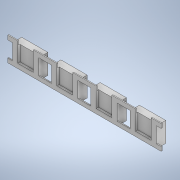
# Autodesk Inventor part: buttons
Saved by Autodesk Inventor 2020 (Build 240168000, 168)
## iProperties
Created: 2022-10-02
Part Number: buttons
Material: Типовые
Document SubType Name: Modeling
Designer: NoName
Density: 1 g/cm^3
Appearance: По умолчанию
Author: NoName
Autodesk Inventor part; units mm, degrees
ref_plane "YZ Plane" through (0, 0, 0) normal (1, 0, 0) x (0, 1, 0)
ref_plane "XZ Plane" through (0, 0, 0) normal (0, 1, 0) x (-1, 0, 0)
ref_plane "XY Plane" through (0, 0, 0) normal (0, 0, 1) x (1, 0, 0)
sketch "Эскиз1" plane through (0, 0, 0) normal (0, 0, 1) x (1, 0, 0)
  line L0 (0, 0) -> (5.7, 0)
  line L1 (5.7, 0) -> (5.7, 4.3)
  line L2 (5.7, 4.3) -> (0, 4.3)
  line L3 (0, 4.3) -> (0, 0)
  line L4 (8.5, 0) -> (14.2, 0)
  line L5 (14.2, 0) -> (14.2, 4.3)
  line L6 (14.2, 4.3) -> (8.5, 4.3)
  line L7 (8.5, 4.3) -> (8.5, 0)
  line L8 (17, 0) -> (22.7, 0)
  line L9 (22.7, 0) -> (22.7, 4.3)
  line L10 (22.7, 4.3) -> (17, 4.3)
  line L11 (17, 4.3) -> (17, 0)
  line L12 (25.5, 0) -> (31.2, 0)
  line L13 (31.2, 0) -> (31.2, 4.3)
  line L14 (31.2, 4.3) -> (25.5, 4.3)
  line L15 (25.5, 4.3) -> (25.5, 0)
  dimension "d0" = 4.3
  dimension "d1" = 5.7
  dimension "d4" = 8.5
  constraints: 32 end point, 2 horizontal, 2 parallel, 1 collinear, 1 perpendicular, 23 other
  measures "d0" distance between parallel lines of L0 L2
  measures "d1" distance between parallel lines of L1 L3
  measures "d4" distance of L0.start L4.start
extrude "Выдавливание1" add sketch "Эскиз1" along normal blind 2.4
sketch "Эскиз2" plane through (0, 0, 2.4) normal (0, 0, 1) x (1, 0, 0)
  line L0 (-1, 4.3) -> (32.2, 4.3)
  line L1 (32.2, 4.3) -> (32.2, 5.2)
  line L2 (32.2, 5.2) -> (-1, 5.2)
  line L3 (-1, 5.2) -> (-1, 4.3)
  line L4 (-1, 0) -> (32.2, 0)
  line L5 (32.2, 0) -> (32.2, 0.9)
  line L6 (32.2, 0.9) -> (-1, 0.9)
  line L7 (-1, 0.9) -> (-1, 0)
  line L8 (5.7, 4.3) -> (0, 4.3) projected
  line L9 (0, 4.3) -> (5.7, 4.3)
  line L10 (5.7, 4.3) -> (5.7, 4.3)
  line L11 (5.7, 4.3) -> (0, 4.3)
  line L12 (0, 4.3) -> (0, 4.3)
  line L13 (14.2, 4.3) -> (8.5, 4.3) projected
  line L14 (8.5, 4.3) -> (14.2, 4.3)
  line L15 (14.2, 4.3) -> (14.2, 4.3)
  line L16 (14.2, 4.3) -> (8.5, 4.3)
  line L17 (8.5, 4.3) -> (8.5, 4.3)
  line L18 (17, 4.3) -> (22.7, 4.3)
  line L19 (22.7, 4.3) -> (22.7, 4.3)
  line L20 (22.7, 4.3) -> (17, 4.3)
  line L21 (17, 4.3) -> (17, 4.3)
  line L22 (31.2, 4.3) -> (25.5, 4.3) projected
  line L23 (25.5, 4.3) -> (31.2, 4.3)
  line L24 (31.2, 4.3) -> (31.2, 4.3)
  line L25 (31.2, 4.3) -> (25.5, 4.3)
  line L26 (25.5, 4.3) -> (25.5, 4.3)
  line L27 (0, 4.3) -> (0, 0) projected
  line L28 (31.2, 0) -> (31.2, 4.3) projected
  point P0 (31.2, 0.9)
  point P1 (0, 0.9)
  point P2 (25.5, 4.8)
  point P3 (17, 4.8)
  point P4 (0, 4.8)
  point P5 (8.5, 4.8)
  dimension "d11" = 0.9
  dimension "d12" = 0
  dimension "d13" = 0.9
  dimension "d14" = 1
  dimension "d15" = 1
  constraints: 48 end point, 12 equal length, 6 horizontal, 6 perpendicular, 4 point on line, 2 vertical alignment, 1 coincident, 1 horizontal alignment
  measures "d11" distance between parallel lines of L4 L6
  measures "d12" distance between parallel lines of L8 L0
  measures "d13" distance between parallel lines of L2 L0
  measures "d14" distance between parallel lines of L3 L27
  measures "d15" distance between parallel lines of L28 L1
extrude "Выдавливание2" add sketch "Эскиз2" against normal blind 0.2 contours L3 L2 L1 L0 | L27 L4 L7 L6 | L6 L28 L4 L27 | L6 L5 L4 L28
sketch "Эскиз3" plane through (0, 0, 2.4) normal (0, 0, 1) x (1, 0, 0)
  line L0 (32.2, 5.2) -> (-1, 5.2) projected
  line L1 (1.15, 1) -> (4.55, 1)
  line L2 (4.55, 1) -> (4.55, 5.2)
  line L3 (4.55, 5.2) -> (1.15, 5.2)
  line L4 (1.15, 5.2) -> (1.15, 1)
  line L5 (0, 4.3) -> (5.7, 4.3) projected
  line L6 (9.65, 1) -> (13.05, 1)
  line L7 (13.05, 1) -> (13.05, 5.2)
  line L8 (13.05, 5.2) -> (9.65, 5.2)
  line L9 (9.65, 5.2) -> (9.65, 1)
  line L10 (18.15, 1) -> (21.55, 1)
  line L11 (21.55, 1) -> (21.55, 5.2)
  line L12 (21.55, 5.2) -> (18.15, 5.2)
  line L13 (18.15, 5.2) -> (18.15, 1)
  line L14 (26.65, 1) -> (30.05, 1)
  line L15 (30.05, 1) -> (30.05, 5.2)
  line L16 (30.05, 5.2) -> (26.65, 5.2)
  line L17 (26.65, 5.2) -> (26.65, 1)
  point P0 (0, 0)
  point P1 (2.85, 4.3)
  point P2 (2.85, 1)
  point P3 (11.35, 1)
  point P4 (11.35, 4.3)
  point P5 (19.85, 1)
  point P6 (19.85, 4.3)
  point P7 (28.35, 1)
  point P8 (28.35, 4.3)
  point P9 (13.05, 5.2)
  point P10 (21.55, 5.2)
  point P11 (30.05, 5.2)
  dimension "d18" = 3.4
  dimension "d19" = 4.2
  dimension "d22" = 8.5
  constraints: 32 end point, 2 horizontal, 2 midpoint, 2 parallel, 1 perpendicular, 1 point on line, 1 vertical alignment, 30 other
  measures "d18" distance between parallel lines of L2 L4
  measures "d19" distance between parallel lines of L0 L1
  measures "d22" distance of L1.start L6.start
extrude "Выдавливание3" cut sketch "Эскиз3" against normal blind 0.5
chamfer "Фаска1" distance 0.4 angle 45 16 edges at (2.85, 4.3, 0) (0, 2.15, 0) (2.85, 0, 0) (5.7, 2.15, 0) (8.5, 2.15, 0) (11.35, 4.3, 0) (14.2, 2.15, 0) (11.35, 0, 0) (19.85, 0, 0) (17, 2.15, 0) (19.85, 4.3, 0) (22.7, 2.15, 0) (25.5, 2.15, 0) (28.35, 4.3, 0) (31.2, 2.15, 0) (28.35, 0, 0)
